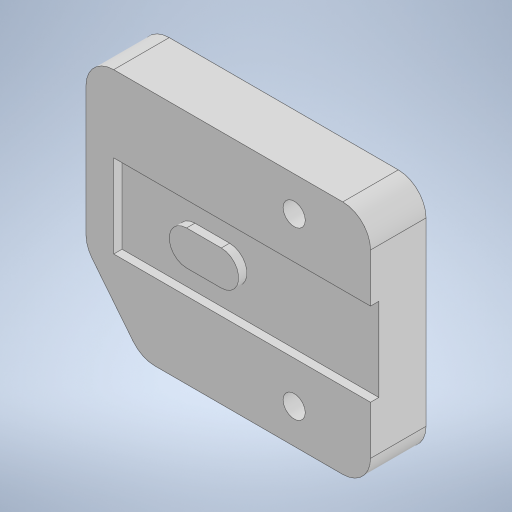
# Autodesk Inventor part: cutter_holder-2
Saved by Autodesk Inventor 2024 (Build 280153000, 153)
## iProperties
Created: 2025-06-13
Part Number: cutter_holder-2
Material: 一般
Document SubType Name: Modeling
Designer: 1412z
Density: 1 g/cm^3
Appearance: 既定
Author: 1412z
Autodesk Inventor part; units mm, degrees
ref_plane "YZ Plane" through (0, 0, 0) normal (1, 0, 0) x (0, 1, 0)
ref_plane "XZ Plane" through (0, 0, 0) normal (0, 1, 0) x (-1, 0, 0)
ref_plane "XY Plane" through (0, 0, 0) normal (0, 0, 1) x (1, 0, 0)
sketch "スケッチ1" plane through (0, 0, 0) normal (0, 0, 1) x (1, 0, 0)
  line L0 (0, 0) -> (-20.5, 0)
  line L1 (-20.5, 0) -> (-20.5, -17)
  line L2 (-20.5, -17) -> (0, -17)
  line L3 (0, -17) -> (0, 0)
  dimension "d0" = 20.5
  dimension "d1" = 17
  constraints: 8 end point, 2 parallel, 1 horizontal, 1 perpendicular
  measures "d0" distance of L2.end L1.end
  measures "d1" distance of L1.end L0.end
extrude "押し出し1" add sketch "スケッチ1" along normal blind 4
sketch "スケッチ2" plane through (0, 0, 4) normal (0, 0, 1) x (1, 0, 0)
  circle A0 centre (-5.5, -2.5) radius 0.8
  circle A1 centre (-5.5, -14.5) radius 0.8
  point P0 (0, 0)
  dimension "d4" = 1.6
  dimension "d5" = 1.6
  constraints: 2 centre point
  measures "d4" diameter of A0
  measures "d5" diameter of A1
extrude "押し出し2" cut sketch "スケッチ2" against normal blind 4
sketch "スケッチ3" plane through (0, 0, 4) normal (0, 0, 1) x (1, 0, 0)
  line L0 (0, -17) -> (0, 0) projected
  line L1 (0, -8.5) -> (0, -11.5)
  line L2 (0, -11.5) -> (-18.5, -11.5)
  line L3 (-20.5, 0) -> (-20.5, -17) projected
  line L4 (-18.5, -11.5) -> (-18.5, -5.5)
  line L5 (-18.5, -5.5) -> (0, -5.5)
  line L6 (0, -5.5) -> (0, -8.5)
  point P0 (0, -5.5)
  dimension "d8" = 3
  dimension "d9" = 18.5
  dimension "d10" = 6
  constraints: 10 end point, 4 perpendicular, 2 point on line, 1 midpoint
  measures "d8" distance of L1.start L1.end
  measures "d9" distance of L1.end L2.end
  measures "d10" distance of L2.end L4.end
extrude "押し出し3" cut sketch "スケッチ3" against normal blind 0.6
sketch "スケッチ4" plane through (0, 0, 3.4) normal (0, 0, 1) x (1, 0, 0)
  circle A0 centre (-13.25, -8.5) radius 1.25
  circle A1 centre (-10.75, -8.5) radius 1.25
  line L0 (-10.75, -9.75) -> (-13.25, -9.75)
  line L1 (-10.75, -7.25) -> (-13.25, -7.25)
  line L2 (-18.5, -11.5) -> (-18.5, -5.5) projected
  point P0 (0, 0)
  dimension "d13" = 2.5
  dimension "d16" = 5.25
  dimension "d17" = 2.5
  constraints: 4 end point, 4 point on circle, 2 centre point, 2 tangent, 1 parallel
  measures "d13" diameter of A0
  measures "d16" distance from line of L2 A0.centre
  measures "d17" distance of L1.start L1.end
extrude "押し出し4" add sketch "スケッチ4" along normal blind 0.6
sketch "スケッチ5" plane through (0, 0, 4) normal (0, 0, 1) x (1, 0, 0)
  line L0 (-20.5, -17) -> (0, -17) projected
  line L1 (-20.5, -17) -> (-20.5, -12)
  line L2 (-20.5, -17) -> (-16.5, -17)
  line L3 (-16.5, -17) -> (-20.5, -12)
  line L4 (-20.5, 0) -> (-20.5, -5)
  line L5 (0, 0) -> (-20.5, 0) projected
  point P0 (-16.5, 0)
  dimension "d18" = 5
  dimension "d19" = 4
  dimension "d20" = 5
  dimension "d21" = 4
  constraints: 8 end point, 2 point on line
  measures "d18" distance of L0.start L1.end
  measures "d19" distance of L0.start L2.end
  measures "d20" distance of L4.start L4.end
  measures "d21" distance of L4.start point (-16.5, 0)
extrude "押し出し5" cut sketch "スケッチ5" against normal blind 10
fillet "フィレット1" radius 2 4 edges at (-20.5, -12, 2) (-16.5, -17, 2) (0, -17, 2) (0, 0, 2)
fillet "フィレット2" radius 2 1 edges at (-20.5, 0, 2)
